Autodesk Inventor part; units mm, degrees
(part 3 of 3)
  spline S315 degree 2 poles (6.6876, 44.1549) (5.7783, 44.1549) (4.927, 45.5678) (4.927, 47.0164) knots 0 0 0 1 2 2 2
  spline S316 degree 2 poles (4.927, 47.0164) (4.927, 48.505) (5.7872, 49.8823) (6.6876, 49.8823) knots 0 0 0 1 2 2 2
  spline S317 degree 2 poles (6.6876, 49.8823) (7.5923, 49.8823) (8.4436, 48.456) (8.4436, 47.0208) knots 0 0 0 1 2 2 2
  spline S318 degree 2 poles (7.4987, 45.345) (7.6057, 45.6169) (7.6949, 46.4548) (7.6949, 47.0208) knots 0 0 0 1 2 2 2
  spline S319 degree 2 poles (7.6949, 47.0208) (7.6949, 47.5869) (7.6057, 48.4203) (7.4943, 48.7011) knots 0 0 0 1 2 2 2
  spline S320 degree 2 poles (7.4943, 48.7011) (7.3829, 48.9819) (6.9951, 49.2716) (6.6876, 49.2716) knots 0 0 0 1 2 2 2
  spline S321 degree 2 poles (6.6876, 49.2716) (6.38, 49.2716) (5.9833, 48.9819) (5.8675, 48.6922) knots 0 0 0 1 2 2 2
  spline S322 degree 2 poles (5.8675, 48.6922) (5.756, 48.4114) (5.6758, 47.5557) (5.6758, 47.0164) knots 0 0 0 1 2 2 2
  spline S323 degree 2 poles (5.6758, 47.0164) (5.6758, 46.437) (5.7471, 45.6614) (5.863, 45.3583) knots 0 0 0 1 2 2 2
  spline S324 degree 2 poles (5.863, 45.3583) (5.97, 45.0731) (6.3667, 44.7656) (6.6876, 44.7656) knots 0 0 0 1 2 2 2
  spline S325 degree 2 poles (6.6876, 44.7656) (6.9906, 44.7656) (7.3873, 45.0553) (7.4987, 45.345) knots 0 0 0 1 2 2 2
  spline S326 degree 2 poles (4.2735, 17.0475) (4.2735, 15.5677) (3.4133, 14.1816) (2.5174, 14.1816) knots 0 0 0 1 2 2 2
  spline S327 degree 2 poles (2.5174, 14.1816) (1.6082, 14.1816) (0.7569, 15.5945) (0.7569, 17.043) knots 0 0 0 1 2 2 2
  spline S328 degree 2 poles (0.7569, 17.043) (0.7569, 18.5317) (1.6171, 19.9089) (2.5174, 19.9089) knots 0 0 0 1 2 2 2
  spline S329 degree 2 poles (2.5174, 19.9089) (3.4222, 19.9089) (4.2735, 18.4826) (4.2735, 17.0475) knots 0 0 0 1 2 2 2
  spline S330 degree 2 poles (3.3286, 15.3716) (3.4356, 15.6435) (3.5247, 16.4814) (3.5247, 17.0475) knots 0 0 0 1 2 2 2
  spline S331 degree 2 poles (3.5247, 17.0475) (3.5247, 17.6135) (3.4356, 18.447) (3.3241, 18.7278) knots 0 0 0 1 2 2 2
  spline S332 degree 2 poles (3.3241, 18.7278) (3.2127, 19.0086) (2.825, 19.2983) (2.5174, 19.2983) knots 0 0 0 1 2 2 2
  spline S333 degree 2 poles (2.5174, 19.2983) (2.2099, 19.2983) (1.8132, 19.0086) (1.6973, 18.7188) knots 0 0 0 1 2 2 2
  spline S334 degree 2 poles (1.6973, 18.7188) (1.5859, 18.4381) (1.5057, 17.5823) (1.5057, 17.043) knots 0 0 0 1 2 2 2
  spline S335 degree 2 poles (1.5057, 17.043) (1.5057, 16.4636) (1.577, 15.6881) (1.6929, 15.385) knots 0 0 0 1 2 2 2
  spline S336 degree 2 poles (1.6929, 15.385) (1.7998, 15.0997) (2.1965, 14.7922) (2.5174, 14.7922) knots 0 0 0 1 2 2 2
  spline S337 degree 2 poles (2.5174, 14.7922) (2.8205, 14.7922) (3.2172, 15.0819) (3.3286, 15.3716) knots 0 0 0 1 2 2 2
  line L203 (4.3195, 33.9241) -> (0.9276, 33.9241)
  line L204 (0.9276, 33.9241) -> (0.9276, 34.7041)
  spline S338 degree 2 poles (0.9276, 34.7041) (1.2931, 35.0472) (1.9438, 35.6846) (2.2558, 36.0278) knots 0 0 0 1 2 2 2
  spline S339 degree 2 poles (2.2558, 36.0278) (2.8843, 36.7186) (3.3434, 37.5477) (3.3434, 37.9889) knots 0 0 0 1 2 2 2
  spline S340 degree 2 poles (3.3434, 37.9889) (3.3434, 38.2207) (3.2007, 38.5683) (3.0715, 38.6797) knots 0 0 0 1 2 2 2
  spline S341 degree 2 poles (3.0715, 38.6797) (2.9422, 38.7912) (2.6035, 38.9026) (2.3985, 38.9026) knots 0 0 0 1 2 2 2
  spline S342 degree 2 poles (2.3985, 38.9026) (2.2024, 38.9026) (1.8012, 38.8045) (1.6185, 38.7288) knots 0 0 0 1 2 2 2
  spline S343 degree 2 poles (1.6185, 38.7288) (1.4625, 38.6664) (1.1728, 38.4881) (1.0836, 38.4257) knots 0 0 0 1 2 2 2
  line L205 (1.0836, 38.4257) -> (1.0435, 38.4257)
  line L206 (1.0435, 38.4257) -> (1.0435, 39.2101)
  spline S344 degree 2 poles (1.0435, 39.2101) (1.2708, 39.3216) (2.0865, 39.54) (2.452, 39.54) knots 0 0 0 1 2 2 2
  spline S345 degree 2 poles (2.452, 39.54) (3.223, 39.54) (4.0921, 38.7243) (4.0921, 38.029) knots 0 0 0 1 2 2 2
  spline S346 degree 2 poles (4.0921, 38.029) (4.0921, 37.7037) (3.9406, 37.1599) (3.8069, 36.9281) knots 0 0 0 1 2 2 2
  spline S347 degree 2 poles (3.8069, 36.9281) (3.6732, 36.6874) (3.2854, 36.215) (3.0715, 35.9877) knots 0 0 0 1 2 2 2
  spline S348 degree 2 poles (3.0715, 35.9877) (2.7238, 35.6088) (1.8725, 34.7977) (1.6185, 34.5614) knots 0 0 0 1 2 2 2
  line L207 (1.6185, 34.5614) -> (4.3195, 34.5614)
  line L208 (4.3195, 34.5614) -> (4.3195, 33.9241)
  spline S349 degree 2 poles (8.4779, 36.6741) (8.4779, 35.1943) (7.6177, 33.8082) (6.7218, 33.8082) knots 0 0 0 1 2 2 2
  spline S350 degree 2 poles (6.7218, 33.8082) (5.8126, 33.8082) (4.9613, 35.2211) (4.9613, 36.6696) knots 0 0 0 1 2 2 2
  spline S351 degree 2 poles (4.9613, 36.6696) (4.9613, 38.1583) (5.8215, 39.5355) (6.7218, 39.5355) knots 0 0 0 1 2 2 2
  spline S352 degree 2 poles (6.7218, 39.5355) (7.6266, 39.5355) (8.4779, 38.1092) (8.4779, 36.6741) knots 0 0 0 1 2 2 2
  spline S353 degree 2 poles (7.533, 34.9982) (7.64, 35.2701) (7.7291, 36.108) (7.7291, 36.6741) knots 0 0 0 1 2 2 2
  spline S354 degree 2 poles (7.7291, 36.6741) (7.7291, 37.2401) (7.64, 38.0736) (7.5285, 38.3544) knots 0 0 0 1 2 2 2
  spline S355 degree 2 poles (7.5285, 38.3544) (7.4171, 38.6352) (7.0293, 38.9249) (6.7218, 38.9249) knots 0 0 0 1 2 2 2
  spline S356 degree 2 poles (6.7218, 38.9249) (6.4143, 38.9249) (6.0176, 38.6352) (5.9017, 38.3455) knots 0 0 0 1 2 2 2
  spline S357 degree 2 poles (5.9017, 38.3455) (5.7903, 38.0647) (5.7101, 37.2089) (5.7101, 36.6696) knots 0 0 0 1 2 2 2
  spline S358 degree 2 poles (5.7101, 36.6696) (5.7101, 36.0902) (5.7814, 35.3147) (5.8973, 35.0116) knots 0 0 0 1 2 2 2
  spline S359 degree 2 poles (5.8973, 35.0116) (6.0042, 34.7263) (6.4009, 34.4188) (6.7218, 34.4188) knots 0 0 0 1 2 2 2
  spline S360 degree 2 poles (6.7218, 34.4188) (7.0249, 34.4188) (7.4216, 34.7085) (7.533, 34.9982) knots 0 0 0 1 2 2 2
  point P0 (190.5653, 91.5)
  point P1 (8.4853, 17.25)
  dimension "d94" = 1
  constraints: 14 end point, 3 midpoint, 2 parallel, 2 perpendicular, 2 point on line, 1 horizontal, 30 other
  measures "d94" distance of L61.end L62.end
extrude "Extrusion14" add sketch "Skizze14" along normal blind 1 contours L61 L62 L63 L67 | L68 L69 L70 L71 L72 L73 S0 L74 L75 L76 L77 | S1 S2 S3 S4 S5 S6 S7 L78 L79 S8 S9 S10 S11 S12 | S20 S21 S22 S23 | L80 L81 L82 L83 L84 L85 S32 L86 L87 L88 L89 | S33 S34 S35 L90 L91 S36 S37 S38 S39 S40 S41 S42 L92 L93 L94 L95 L96 S43 S44 S45 | S46 S47 S48 S49 | L97 L98 L99 L100 L101 L102 S58 L103 L104 L105 L106 | S59 S60 L107 L108 S61 S62 S63 S64 L109 S65 S66 S67 S68 S69 L110 L111 S70 S71 S72 S73 S74 L112 L113 L114 S75 S76 S77 | S78 S79 S80 S81 | L115 L116 L117 L118 L119 L120 S90 L121 L122 L123 L124 | L125 L126 S91 S92 S93 S94 S95 S96 L127 L128 S97 S98 S99 S100 S101 L129 L130 | S102 S103 S104 S105 | L131 L132 L133 L134 L135 L136 S114 L137 L138 L139 L140 | L141 L142 L143 L144 L145 L146 S115 L147 L148 L149 L150 | S116 S117 S118 S119 | L151 L152 L153 L154 L155 L156 S128 L157 L158 L159 L160 | S129 S130 S131 S132 | S141 S142 S143 S144 | S153 S154 S155 S156 S157 S158 S159 L161 L162 S160 S161 S162 S163 S164 | S172 S173 S174 S175 | S184 S185 S186 L163 S187 S188 S189 S190 L164 S191 S192 | S203 S204 S205 S206 | L165 L166 L167 L168 L169 L170 L171 | S215 S216 S217 S218 | S227 S228 S229 S230 S231 S232 S233 L172 L173 S234 S235 S236 S237 S238 | S246 S247 S248 S249 | S258 S259 S260 L174 L175 S261 S262 S263 S264 S265 S266 S267 L176 L177 L178 L179 L180 S268 S269 S270 | S271 S272 S273 S274 | L181 L182 L183 L184 L185 L186 L187 L188 L189 L190 L191 | S283 S284 S285 S286 | S295 S296 L195 L196 S297 S298 S299 S300 L197 S301 S302 S303 S304 S305 L198 L199 S306 S307 S308 S309 S310 L200 L201 L202 S311 S312 S313 | S314 S315 S316 S317 | S326 S327 S328 S329 | L203 L204 S338 S339 S340 S341 S342 S343 L205 L206 S344 S345 S346 S347 S348 L207 L208 | S349 S350 S351 S352
sketch "Skizze17" plane through (-65, -62, 24) normal (0, -1, 0) x (1, 0, 0)
  line L0 (-5, 0) -> (-5, 156.5)
  line L1 (-5, 156.5) -> (-6, 157.5) projected
  line L2 (-5, 156.5) -> (-6, 157.5)
  line L3 (-13.5, 165) -> (-22, 156.5) projected
  line L4 (-6, 157.5) -> (-13.5, 165)
  line L5 (-13.5, 165) -> (-22, 156.5)
  line L6 (-5, 0) -> (-22, 0) projected
  line L7 (-22, 156.5) -> (-22, 0)
  line L8 (-22, 0) -> (-5, 0)
  line L9 (135, 0) -> (135, 156.5)
  line L10 (136, 157.4) -> (135, 156.5) projected
  line L11 (135, 156.5) -> (136, 157.4)
  line L12 (143.9474, 164.5526) -> (136, 157.4) projected
  line L13 (136, 157.4) -> (143.9474, 164.5526)
  line L14 (152, 0) -> (152, 156.5) projected
  line L15 (143.9474, 164.5526) -> (152, 156.5)
  line L16 (136, 0) -> (152, 0) projected
  line L17 (152, 156.5) -> (152, 0)
  line L18 (152, 0) -> (135, 0)
  point P0 (65, -24)
  constraints: 25 end point, 4 collinear, 4 perpendicular, 1 vertical
extrude "Extrusion15" add sketch "Skizze17" against normal blind 3
sketch "Skizze18" plane through (-71, -86.5, 181.5) normal (1, 0, 0) x (0, 0, -1)
  line L0 (-5, 24.5) -> (1, 24.5) projected
  line L1 (0, 24.5) -> (0, 0) projected
  line L2 (0, 24.5) -> (0, 0)
  line L3 (157.5, 0) -> (160.5, 0) projected
  line L4 (0, 0) -> (157.5, 0)
  line L5 (157.5, 24.5) -> (160.5, 24.5) projected
  line L6 (157.5, 0) -> (157.5, 24.5)
  line L7 (-5, 24.5) -> (0, 24.5) projected
  line L8 (157.5, 24.5) -> (0, 24.5)
  point P0 (181.5, 86.5)
  point P1 (1, 24.5)
  constraints: 8 end point, 3 collinear, 1 perpendicular, 1 point on line
extrude "Extrusion16" add sketch "Skizze18" against normal blind 3
sketch "Skizze20" plane through (71, -86.5, 181.4) normal (-1, 0, 0) x (0, 0, 1)
  line L0 (5.1, 24.5) -> (0, 24.5) projected
  line L1 (0, 0) -> (0, 24.5) projected
  line L2 (0, 24.5) -> (0, 0)
  line L3 (-157.4, 0) -> (-157.4, 24.5) projected
  line L4 (0, 0) -> (-157.4, 0)
  line L5 (-157.4, 0) -> (-157.4, 24.5)
  line L6 (-157.4, 24.5) -> (0, 24.5)
  point P0 (-181.4, 86.5)
  constraints: 8 end point, 3 perpendicular, 1 collinear
extrude "Extrusion17" add sketch "Skizze20" against normal blind 3
sketch "Skizze30" plane through (89, -91.5, 0) normal (1, 0, 0) x (0, 0, -1)
  line L0 (0, 0) -> (0, 183) projected
  line L1 (-24, 181) -> (-24, 32.5) projected
  line L2 (0, 183) -> (-24, 183)
  line L3 (-24, 183) -> (-24, 159)
  line L4 (-24, 159) -> (0, 159)
  line L5 (0, 159) -> (0, 183)
  line L6 (-180.5, 183) -> (-180.5, 169.25) projected
  line L7 (-180.5, 183) -> (-156.5, 183)
  line L8 (-156.5, 183) -> (-156.5, 159)
  line L9 (-156.5, 159) -> (-180.5, 159)
  line L10 (-180.5, 159) -> (-180.5, 183)
  line L11 (-24, 0) -> (-180.5, 0) projected
  line L12 (-180.5, 0) -> (-156.5, 0)
  line L13 (-156.5, 0) -> (-156.5, 24)
  line L14 (-156.5, 24) -> (-180.5, 24)
  line L15 (-180.5, 24) -> (-180.5, 0)
  line L16 (0, 0) -> (-24, 0)
  line L17 (-24, 0) -> (-24, 24)
  line L18 (-24, 24) -> (0, 24)
  line L19 (0, 24) -> (0, 0)
  point P0 (0, 91.5)
  point P1 (0, 24)
  dimension "d140" = 24
  dimension "d141" = 24
  dimension "d142" = 24
  dimension "d143" = 24
  dimension "d144" = 24
  dimension "d145" = 24
  dimension "d146" = 24
  constraints: 32 end point, 8 parallel, 4 horizontal, 4 perpendicular, 1 point on line
  measures "d140" distance of L0.end L2.end
  measures "d141" distance of L3.end L2.end
  measures "d142" distance of L6.start L7.end
  measures "d143" distance of L13.end L14.end
  measures "d144" distance of L12.end L13.end
  measures "d145" distance of L17.end L18.end
  measures "d146" distance of L16.end L17.end
extrude "Extrusion20" add sketch "Skizze30" against normal blind 5
sketch "Skizze33" plane through (89, -91.5, 0) normal (1, 0, 0) x (0, 0, -1)
  line L0 (-180.5, 0) -> (-180.5, 183) projected
  line L1 (0, 0) -> (-180.5, 0) projected
  line L2 (0, 183) -> (-180.5, 183) projected
  line L3 (0, 183) -> (-180.5, 183) projected
  line L4 (0, 0) -> (0, 183) projected
  line L5 (-5, 5) -> (-19, 5)
  line L6 (-19, 5) -> (-19, 19)
  line L7 (-19, 19) -> (-5, 19)
  line L8 (-5, 19) -> (-5, 5)
  line L9 (-5, 178) -> (-19, 178)
  line L10 (-19, 178) -> (-19, 164)
  line L11 (-19, 164) -> (-5, 164)
  line L12 (-5, 164) -> (-5, 178)
  line L13 (-175.5, 178) -> (-161.5, 178)
  line L14 (-161.5, 178) -> (-161.5, 164)
  line L15 (-161.5, 164) -> (-175.5, 164)
  line L16 (-175.5, 164) -> (-175.5, 178)
  line L17 (-175.5, 5) -> (-161.5, 5)
  line L18 (-161.5, 5) -> (-161.5, 19)
  line L19 (-161.5, 19) -> (-175.5, 19)
  line L20 (-175.5, 19) -> (-175.5, 5)
  point P0 (0, 91.5)
  point P1 (-32, 183)
  point P2 (-31, 183)
  dimension "d161" = 5
  dimension "d162" = 5
  dimension "d163" = 5
  dimension "d164" = 5
  dimension "d165" = 5
  dimension "d166" = 5
  dimension "d167" = 5
  dimension "d168" = 5
  dimension "d169" = 14
  dimension "d170" = 14
  dimension "d171" = 14
  dimension "d172" = 14
  dimension "d173" = 14
  dimension "d174" = 14
  dimension "d175" = 14
  dimension "d176" = 14
  constraints: 32 end point, 8 parallel, 4 horizontal, 4 perpendicular, 2 point on line
  measures "d161" distance from line of L17.start L0
  measures "d162" distance from line of L1 L17.start
  measures "d163" distance from line of L2 L13.start
  measures "d164" distance from line of L13.start L0
  measures "d165" distance from line of L3 L9.start
  measures "d166" distance from line of L9.start L4
  measures "d167" distance from line of L5.start L1
  measures "d168" distance from line of L5.start L4
  measures "d169" distance of L19.end L17.start
  measures "d170" distance of L18.end L19.end
  measures "d171" distance of L14.end L15.end
  measures "d172" distance of L15.end L13.start
  measures "d173" distance of L9.end L10.end
  measures "d174" distance of L9.start L9.end
  measures "d175" distance of L6.end L7.end
  measures "d176" distance of L5.end L6.end
extrude "Extrusion21" cut sketch "Skizze33" against normal blind 3 contours L5 L6 L7 L8 | L12 L11 L10 L9 | L13 L14 L15 L16 | L20 L19 L18 L17
sketch "Skizze35" plane through (-89, 91.5, 0) normal (0, 1, 0) x (1, 0, 0)
  line L0 (154, -24) -> (24, -24) projected
  line L1 (79, 24) -> (99, 24)
  line L2 (99, 24) -> (99, -24)
  line L3 (99, -24) -> (79, -24)
  line L4 (79, -24) -> (79, 24)
  line L5 (79, 24) -> (99, -24) construction
  line L6 (99, 24) -> (79, -24) construction
  line L7 (78, -24) -> (80, -24)
  line L8 (80, -24) -> (80, 24)
  line L9 (80, 24) -> (78, 24)
  line L10 (78, 24) -> (78, -24)
  line L11 (78, -24) -> (80, 24) construction
  line L12 (80, -24) -> (78, 24) construction
  line L13 (100, -24) -> (98, -24)
  line L14 (98, -24) -> (98, 24)
  line L15 (98, 24) -> (100, 24)
  line L16 (100, 24) -> (100, -24)
  line L17 (13.65, 0) -> (164.35, 0) projected
  line L18 (100, -24) -> (98, 24) construction
  line L19 (98, -24) -> (100, 24) construction
  point P0 (89, 0)
  point P1 (79, 0)
  point P2 (99, 0)
  point P3 (78, 0)
  point P4 (100, 0)
  dimension "d179" = 20
  dimension "d180" = 2
  dimension "d181" = 2
  constraints: 36 end point, 8 midpoint, 6 parallel, 4 point on line, 3 horizontal, 3 perpendicular
  measures "d179" distance of L1.start L1.end
  measures "d180" distance of L14.end L15.end
  measures "d181" distance of L9.end L8.end
extrude "Extrusion22" cut sketch "Skizze35" against normal blind 1 contours L0 L2 L17 L16 | L0 L10 L17 L4
sketch "Skizze36" plane through (-89, 90.5, 0) normal (0, 1, 0) x (1, 0, 0)
  line L0 (78, -24) -> (78, 0) projected
  line L1 (78, 0) -> (79, 0)
  line L2 (79, 0) -> (79, -1)
  line L3 (79, -1) -> (78, -1)
  line L4 (78, -1) -> (78, 0)
  line L5 (13.65, 0) -> (164.35, 0) projected
  line L6 (99, 0) -> (100, 0)
  line L7 (100, 0) -> (100, -1)
  line L8 (100, -1) -> (99, -1)
  line L9 (99, -1) -> (99, 0)
  point P0 (89, 0)
  constraints: 16 end point, 4 parallel, 2 horizontal, 2 perpendicular, 1 point on line
extrude "Extrusion23" cut sketch "Skizze36" against normal blind 20
sketch "Skizze38" plane through (-89, 91.5, 180.5) normal (0, 1, 0) x (1, 0, 0)
  line L0 (24, 156.5) -> (24, 92) projected
  line L1 (154, 156.5) -> (154, 92) projected
  point P0 (89, 180.5)
  dimension "d186" = 130
  measures "d186" distance between parallel lines of L0 L1
sketch "Skizze39" plane through (0, 0, 24) normal (0, 0, 1) x (1, 0, 0)
  circle A0 centre (-60.35, 54) radius 1.7 projected
  circle A1 centre (-60.35, 54) radius 3
  circle A2 centre (0, 54) radius 1.7 projected
  circle A3 centre (0, 54) radius 3
  circle A4 centre (60.35, 54) radius 1.7 projected
  circle A5 centre (60.35, 54) radius 3
  circle A6 centre (60.35, 2.5) radius 1.7 projected
  circle A7 centre (60.35, 2.5) radius 3
  circle A8 centre (-60.35, 2.5) radius 1.7 projected
  circle A9 centre (-60.35, 2.5) radius 3
  circle A10 centre (-60.35, -49) radius 1.7 projected
  circle A11 centre (-60.35, -49) radius 3
  circle A12 centre (0, -49) radius 1.7 projected
  circle A13 centre (0, -49) radius 3
  circle A14 centre (60.35, -49) radius 1.7 projected
  circle A15 centre (60.35, -49) radius 3
  point P0 (0, 0)
  dimension "d188" = 6
  dimension "d189" = 6
  dimension "d190" = 6
  dimension "d191" = 6
  dimension "d192" = 6
  dimension "d193" = 6
  dimension "d194" = 6
  dimension "d195" = 6
  constraints: 8 centre point, 8 coincident
  measures "d188" diameter of A15
  measures "d189" diameter of A13
  measures "d190" diameter of A11
  measures "d191" diameter of A9
  measures "d192" diameter of A1
  measures "d193" diameter of A3
  measures "d194" diameter of A5
  measures "d195" diameter of A7
extrude "Extrusion24" cut sketch "Skizze39" against normal blind 20 contours A0 | A1 | A3 | A4 | A5 | A6 | A7 | A8 | A9 | A11 | A12 | A13 | A14 | A15
sketch "Skizze40" plane through (0, 0, 0) normal (0, 0, -1) x (-1, 0, 0)
  line L0 (-89, -91.5) -> (-89, 91.5) projected
  line L1 (89, 91.5) -> (89, -91.5) projected
  line L2 (-89, 91.5) -> (89, 91.5)
  line L3 (89, 91.5) -> (89, -91.5)
  line L4 (89, -91.5) -> (-89, -91.5)
  line L5 (-89, -91.5) -> (-89, 91.5)
  point P0 (0, 0)
  constraints: 8 end point, 2 parallel, 1 horizontal, 1 perpendicular
extrude "Extrusion25" cut sketch "Skizze40" against normal blind 24
sketch "Skizze41" plane through (77, 91.5, 192.5) normal (0, 0, -1) x (0, -1, 0)
  line L0 (0, 166) -> (0, 154) projected
  line L1 (183, 12) -> (183, -12) projected
  line L2 (0, 166) -> (183, 166)
  line L3 (183, 166) -> (183, -12)
  line L4 (183, -12) -> (0, -12)
  line L5 (0, -12) -> (0, 166)
  point P0 (91.5, 77)
  constraints: 8 end point, 2 parallel, 1 horizontal, 1 perpendicular
extrude "Extrusion26" cut sketch "Skizze41" against normal mid plane 24
sketch "Skizze42" plane through (0, 0, 24) normal (0, 0, -1) x (-1, 0, 0)
  line L0 (-87, 89.5) -> (-70, 89.5) projected
  line L1 (-70, -59) -> (-87, -59) projected
  line L2 (-87, 89.5) -> (-70, 89.5)
  line L3 (-70, 89.5) -> (-70, -59)
  line L4 (-70, -59) -> (-87, -59)
  line L5 (-87, -59) -> (-87, 89.5)
  line L6 (-87, -62) -> (-87, -67.5) projected
  line L7 (-74, -62) -> (-74, -86.5) projected
  line L8 (-87, -62) -> (-74, -62)
  line L9 (-74, -62) -> (-74, -86.5)
  line L10 (-74, -86.5) -> (-87, -86.5)
  line L11 (-87, -86.5) -> (-87, -62)
  line L12 (74, -86.5) -> (74, -62) projected
  line L13 (87, -86.5) -> (87, -62) projected
  line L14 (74, -62) -> (87, -62)
  line L15 (87, -62) -> (87, -86.5)
  line L16 (87, -86.5) -> (74, -86.5)
  line L17 (74, -86.5) -> (74, -62)
  line L18 (70, 89.5) -> (70, -59) projected
  line L19 (87, -59) -> (70, -59) projected
  line L20 (70, 89.5) -> (87, 89.5)
  line L21 (87, 89.5) -> (87, -59)
  line L22 (87, -59) -> (70, -59)
  line L23 (70, -59) -> (70, 89.5)
  point P0 (0, 0)
  constraints: 32 end point, 8 parallel, 4 horizontal, 4 perpendicular
extrude "Extrusion27" add sketch "Skizze42" against normal up to surface (156.5 mm away)
sketch "Skizze43" plane through (89, -91.5, 180.5) normal (1, 0, 0) x (0, 0, -1)
  line L0 (5, 178) -> (19, 178) projected
  line L1 (5, 178) -> (19, 178)
  line L2 (19, 178) -> (19, 164)
  line L3 (19, 164) -> (5, 164)
  line L4 (5, 164) -> (5, 178)
  line L5 (5, 5) -> (5, 19) projected
  line L6 (2, 5) -> (26.5, 5) projected
  line L7 (5, 19) -> (19, 19)
  line L8 (19, 19) -> (19, 5)
  line L9 (19, 5) -> (5, 5)
  line L10 (5, 5) -> (5, 19)
  point P0 (180.5, 91.5)
  constraints: 16 end point, 4 parallel, 2 horizontal, 2 perpendicular, 2 point on line
extrude "Extrusion28" cut sketch "Skizze43" against normal blind 3
ref_plane "Arbeitsebene2" through (0, 0, 29) normal (0, 0, -1) x (-1, 0, 0)
sketch "Skizze44" plane through (0, 0, 29) normal (0, 0, -1) x (-1, 0, 0)
  line L0 (-84.85, 73.1454) -> (-82, 74.7909)
  line L1 (-84.85, 69.8546) -> (-84.85, 73.1454)
  line L2 (-82, 74.7909) -> (-79.15, 73.1454)
  line L3 (-82, 68.2091) -> (-84.85, 69.8546)
  line L4 (-79.15, 73.1454) -> (-79.15, 69.8546)
  line L5 (-79.15, 69.8546) -> (-82, 68.2091)
  line L6 (-82, 74.7909) -> (-96.75, 74.7909)
  line L7 (-82, 68.2091) -> (-96.75, 68.2091)
  line L8 (-96.75, 74.7909) -> (-96.75, 68.2091)
  line L9 (-89, 91.5) -> (-65, 91.5) construction
  line L10 (-82, 91.5) -> (-82, -91.5) construction
  line L11 (-65, -91.5) -> (-89, -91.5) construction
  line L12 (-89, -91.5) -> (-89, 91.5) construction
  line L13 (-65, -62) -> (-65, 91.5) construction
  line L14 (-79.15, 33.1454) -> (-79.15, 29.8546)
  line L15 (-82, 34.7909) -> (-79.15, 33.1454)
  line L16 (-79.15, 29.8546) -> (-82, 28.2091)
  line L17 (-82, 28.2091) -> (-84.85, 29.8546)
  line L18 (-84.85, 29.8546) -> (-84.85, 33.1454)
  line L19 (-84.85, 33.1454) -> (-82, 34.7909)
  line L20 (-82, 34.7909) -> (-96.75, 34.7909)
  line L21 (-82, 28.2091) -> (-96.75, 28.2091)
  line L22 (-96.75, 34.7909) -> (-96.75, 28.2091)
  line L23 (-82, -8.2091) -> (-79.15, -9.8546)
  line L24 (-79.15, -9.8546) -> (-79.15, -13.1454)
  line L25 (-79.15, -13.1454) -> (-82, -14.7909)
  line L26 (-82, -14.7909) -> (-84.85, -13.1454)
  line L27 (-84.85, -9.8546) -> (-82, -8.2091)
  line L28 (-84.85, -13.1454) -> (-84.85, -9.8546)
  line L29 (-82, -14.7909) -> (-96.75, -14.7909)
  line L30 (-82, -8.2091) -> (-96.75, -8.2091)
  line L31 (-96.75, -8.2091) -> (-96.75, -14.7909)
  line L32 (-82, -48.2091) -> (-79.15, -49.8546)
  line L33 (-79.15, -49.8546) -> (-79.15, -53.1454)
  line L34 (-79.15, -53.1454) -> (-82, -54.7909)
  line L35 (-82, -54.7909) -> (-84.85, -53.1454)
  line L36 (-84.85, -49.8546) -> (-82, -48.2091)
  line L37 (-84.85, -53.1454) -> (-84.85, -49.8546)
  line L38 (-82, -54.7909) -> (-96.75, -54.7909)
  line L39 (-82, -48.2091) -> (-96.75, -48.2091)
  line L40 (-96.75, -48.2091) -> (-96.75, -54.7909)
  line L41 (0, 91.5) -> (0, -95.2854)
  line L42 (79.15, 73.1454) -> (79.15, 69.8546)
  line L43 (82, 74.7909) -> (79.15, 73.1454)
  line L44 (79.15, 69.8546) -> (82, 68.2091)
  line L45 (82, 68.2091) -> (84.85, 69.8546)
  line L46 (84.85, 69.8546) -> (84.85, 73.1454)
  line L47 (84.85, 73.1454) -> (82, 74.7909)
  line L48 (82, 74.7909) -> (96.75, 74.7909)
  line L49 (82, 68.2091) -> (96.75, 68.2091)
  line L50 (96.75, 74.7909) -> (96.75, 68.2091)
  line L51 (94, 91.5) -> (70, 91.5) construction
  line L52 (82, 91.5) -> (82, -91.5) construction
  line L53 (70, -91.5) -> (94, -91.5) construction
  line L54 (94, -91.5) -> (94, 91.5) construction
  line L55 (70, -62) -> (70, 91.5) construction
  line L56 (82, 34.7909) -> (79.15, 33.1454)
  line L57 (79.15, 33.1454) -> (79.15, 29.8546)
  line L58 (79.15, 29.8546) -> (82, 28.2091)
  line L59 (82, 28.2091) -> (84.85, 29.8546)
  line L60 (84.85, 33.1454) -> (82, 34.7909)
  line L61 (84.85, 29.8546) -> (84.85, 33.1454)
  line L62 (82, 28.2091) -> (96.75, 28.2091)
  line L63 (82, 34.7909) -> (96.75, 34.7909)
  line L64 (96.75, 34.7909) -> (96.75, 28.2091)
  line L65 (82, -14.7909) -> (84.85, -13.1454)
  line L66 (82, -8.2091) -> (96.75, -8.2091)
  line L67 (82, -8.2091) -> (79.15, -9.8546)
  line L68 (84.85, -9.8546) -> (82, -8.2091)
  line L69 (96.75, -8.2091) -> (96.75, -14.7909)
  line L70 (82, -14.7909) -> (96.75, -14.7909)
  line L71 (84.85, -13.1454) -> (84.85, -9.8546)
  line L72 (79.15, -9.8546) -> (79.15, -13.1454)
  line L73 (79.15, -13.1454) -> (82, -14.7909)
  line L74 (82, -54.7909) -> (84.85, -53.1454)
  line L75 (82, -48.2091) -> (96.75, -48.2091)
  line L76 (82, -48.2091) -> (79.15, -49.8546)
  line L77 (84.85, -49.8546) -> (82, -48.2091)
  line L78 (96.75, -48.2091) -> (96.75, -54.7909)
  line L79 (82, -54.7909) -> (96.75, -54.7909)
  line L80 (84.85, -53.1454) -> (84.85, -49.8546)
  line L81 (79.15, -49.8546) -> (79.15, -53.1454)
  line L82 (79.15, -53.1454) -> (82, -54.7909)
  circle A0 centre (82, 71.5) radius 1.7
  circle A1 centre (82, 31.5) radius 1.7
  circle A2 centre (82, -11.5) radius 1.7
  circle A3 centre (82, -51.5) radius 1.7
  circle A4 centre (-82, -51.5) radius 1.7
  circle A5 centre (-82, -11.5) radius 1.7
  circle A6 centre (-82, 31.5) radius 1.7
  circle A7 centre (-82, 71.5) radius 1.7
  point P0 (0, 0)
  point P1 (-82, 71.5)
  point P2 (-82, 71.5)
  point P3 (-82, -51.5)
  point P4 (-82, -11.5)
  point P5 (-82, 31.5)
  point P6 (-82, -11.5)
  point P7 (-82, -11.5)
  point P8 (-82, -11.5)
  point P9 (-82, -51.5)
  point P10 (82, 71.5)
  point P11 (82, -51.5)
  point P12 (82, -11.5)
  point P13 (82, 31.5)
  point P14 (82, -11.5)
  point P15 (82, -11.5)
  point P16 (82, -11.5)
  point P17 (82, -51.5)
  point P18 (82, -51.5)
  point P19 (82, -51.5)
  point P20 (82, 31.5)
  point P21 (82, -11.5)
  point P22 (82, -51.5)
  point P23 (-82, -51.5)
  point P24 (-82, -11.5)
  point P25 (-82, 31.5)
  point P26 (-82, 71.5)
  point P27 (-82, 71.5)
  dimension "d207" = 5.7
  dimension "d208" = 7
  dimension "d209" = 17
  dimension "d210" = 20
  dimension "d211" = 40
  dimension "d212" = 40
  dimension "d213" = 40
  dimension "d214" = 5.7
  dimension "d215" = 5.7
  dimension "d216" = 5.7
  dimension "d225" = 3.4
  dimension "d226" = 3.4
  dimension "d227" = 3.4
  dimension "d228" = 3.4
  dimension "d229" = 3.4
  dimension "d230" = 3.4
  dimension "d231" = 3.4
  dimension "d232" = 3.4
  dimension "d253" = 0
  dimension "d254" = 0
  constraints: 158 end point, 8 centre point, 8 point on line, 1 coincident, 1 midpoint, 1 parallel, 1 vertical, 52 other
  measures "d207" distance between parallel lines of L4 L1
  measures "d208" distance between parallel lines of L12 L10
  measures "d209" distance between parallel lines of L10 L13
  measures "d210" distance from line of L9 point (-82, 71.5)
  measures "d211" distance of L10.end point (-82, -51.5)
  measures "d212" distance of point (-82, 31.5) point (-82, 71.5)
  measures "d213" distance of point (-82, -51.5) point (-82, -11.5)
  measures "d214" distance between parallel lines of L14 L18
  measures "d215" distance between parallel lines of L24 L28
  measures "d216" distance between parallel lines of L33 L37
  measures "d225" diameter of A0
  measures "d226" diameter of A1
  measures "d227" diameter of A2
  measures "d228" diameter of A3
  measures "d229" diameter of A4
  measures "d230" diameter of A5
  measures "d231" diameter of A6
  measures "d232" diameter of A7
  measures "d253" distance of point (-82, 71.5) point (-82, 71.5)
  measures "d254" distance of point (82, 71.5) point (82, 71.5)
extrude "Extrusion29" cut sketch "Skizze44" against normal blind 2.6 contours L1 L3 L7 L8 L6 L0 | L0 L2 L4 L5 L3 L1 | L14 L16 L17 L18 L19 L15 | L19 L18 L17 L21 L22 L20 | L23 L24 L25 L26 L28 L27 | L27 L28 L26 L29 L31 L30 | L32 L33 L34 L35 L37 L36 | L36 L37 L35 L38 L40 L39 | L43 L47 L46 L45 L44 L42 | L48 L50 L49 L45 L46 L47 | L60 L61 L59 L58 L57 L56 | L63 L64 L62 L59 L61 L60 | L73 L72 L67 L68 L71 L65 | L65 L71 L68 L66 L69 L70 | L82 L81 L76 L77 L80 L74 | L74 L80 L77 L75 L78 L79 | A0 | A1 | A2 | A3 | A4 | A5 | A6 | A7
sketch "Skizze45" plane through (89, -91.5, 180.5) normal (1, 0, 0) x (0, 0, -1)
  line L0 (148.9, 166.2909) -> (151.5, 166.2909) construction
  line L1 (151.5, 159.7091) -> (148.9, 159.7091) construction
  line L2 (148.9, 166.2909) -> (151.5, 159.7091) construction
  line L3 (151.5, 159.7091) -> (151.5, 166.2909) construction
  line L4 (151.5, 166.2909) -> (148.9, 159.7091) construction
  line L5 (148.9, 126.2909) -> (148.9, 124.6454) construction
  line L6 (151.5, 119.7091) -> (148.9, 119.7091) construction
  line L7 (148.9, 126.2909) -> (151.5, 119.7091) construction
  line L8 (148.9, 126.2909) -> (151.5, 126.2909) construction
  line L9 (151.5, 126.2909) -> (148.9, 119.7091) construction
  line L10 (148.9, 83.2909) -> (151.5, 83.2909) construction
  line L11 (151.5, 76.7091) -> (151.5, 78.3546) construction
  line L12 (148.9, 83.2909) -> (151.5, 76.7091) construction
  line L13 (151.5, 81.6454) -> (151.5, 83.2909) construction
  line L14 (151.5, 76.7091) -> (148.9, 76.7091) construction
  line L15 (151.5, 83.2909) -> (148.9, 76.7091) construction
  line L16 (148.9, 43.2909) -> (148.9, 41.6454) construction
  line L17 (151.5, 36.7091) -> (148.9, 36.7091) construction
  line L18 (148.9, 43.2909) -> (151.5, 36.7091) construction
  line L19 (151.5, 43.2909) -> (148.9, 43.2909) construction
  line L20 (151.5, 43.2909) -> (148.9, 36.7091) construction
  circle A0 centre (150.2, 40) radius 0.8
  circle A1 centre (150.2, 80) radius 0.8
  circle A2 centre (150.2, 123) radius 0.8
  circle A3 centre (150.2, 163) radius 0.8
  point P0 (180.5, 91.5)
  dimension "d219" = 1.6
  dimension "d220" = 1.6
  dimension "d221" = 1.6
  dimension "d222" = 1.6
  constraints: 18 end point, 4 centre point, 4 midpoint, 1 vertical
  measures "d219" diameter of A3
  measures "d220" diameter of A2
  measures "d221" diameter of A1
  measures "d222" diameter of A0
extrude "Extrusion30" cut sketch "Skizze45" against normal through all
sketch "Skizze46" plane through (0, 0, 24) normal (0, 0, -1) x (-1, 0, 0)
  line L0 (-79.15, 73.1454) -> (-79.15, 69.8546)
  line L1 (-82, 74.7909) -> (-79.15, 73.1454)
  line L2 (-79.15, 69.8546) -> (-82, 68.2091)
  line L3 (-82, 68.2091) -> (-84.85, 69.8546)
  line L4 (-84.85, 69.8546) -> (-84.85, 73.1454)
  line L5 (-84.85, 73.1454) -> (-82, 74.7909)
  line L6 (-82, 74.7909) -> (-96.75, 74.7909)
  line L7 (-82, 68.2091) -> (-96.75, 68.2091)
  line L8 (-96.75, 74.7909) -> (-96.75, 68.2091)
  line L9 (-94, 91.5) -> (-70, 91.5) construction
  line L10 (-82, 91.5) -> (-82, -91.5) construction
  line L11 (-70, -91.5) -> (-94, -91.5) construction
  line L12 (-94, -91.5) -> (-94, 91.5) construction
  line L13 (-70, -62) -> (-70, 91.5) construction
  line L14 (-82, 34.7909) -> (-79.15, 33.1454)
  line L15 (-79.15, 33.1454) -> (-79.15, 29.8546)
  line L16 (-79.15, 29.8546) -> (-82, 28.2091)
  line L17 (-82, 28.2091) -> (-84.85, 29.8546)
  line L18 (-84.85, 33.1454) -> (-82, 34.7909)
  line L19 (-84.85, 29.8546) -> (-84.85, 33.1454)
  line L20 (-82, 28.2091) -> (-96.75, 28.2091)
  line L21 (-82, 34.7909) -> (-96.75, 34.7909)
  line L22 (-96.75, 34.7909) -> (-96.75, 28.2091)
  line L23 (-82, -14.7909) -> (-84.85, -13.1454)
  line L24 (-82, -8.2091) -> (-96.75, -8.2091)
  line L25 (-82, -8.2091) -> (-79.15, -9.8546)
  line L26 (-84.85, -9.8546) -> (-82, -8.2091)
  line L27 (-96.75, -8.2091) -> (-96.75, -14.7909)
  line L28 (-82, -14.7909) -> (-96.75, -14.7909)
  line L29 (-84.85, -13.1454) -> (-84.85, -9.8546)
  line L30 (-79.15, -9.8546) -> (-79.15, -13.1454)
  line L31 (-79.15, -13.1454) -> (-82, -14.7909)
  line L32 (-82, -54.7909) -> (-84.85, -53.1454)
  line L33 (-82, -48.2091) -> (-96.75, -48.2091)
  line L34 (-82, -48.2091) -> (-79.15, -49.8546)
  line L35 (-84.85, -49.8546) -> (-82, -48.2091)
  line L36 (-96.75, -48.2091) -> (-96.75, -54.7909)
  line L37 (-82, -54.7909) -> (-96.75, -54.7909)
  line L38 (-84.85, -53.1454) -> (-84.85, -49.8546)
  line L39 (-79.15, -49.8546) -> (-79.15, -53.1454)
  line L40 (-79.15, -53.1454) -> (-82, -54.7909)
  line L41 (0, 91.5) -> (0, -95.2854)
  line L42 (79.15, 73.1454) -> (79.15, 69.8546)
  line L43 (82, 74.7909) -> (79.15, 73.1454)
  line L44 (79.15, 69.8546) -> (82, 68.2091)
  line L45 (82, 68.2091) -> (84.85, 69.8546)
  line L46 (84.85, 69.8546) -> (84.85, 73.1454)
  line L47 (84.85, 73.1454) -> (82, 74.7909)
  line L48 (82, 74.7909) -> (96.75, 74.7909)
  line L49 (96.75, 74.7909) -> (96.75, 68.2091)
  line L50 (94, 91.5) -> (70, 91.5) construction
  line L51 (82, 68.2091) -> (96.75, 68.2091)
  line L52 (82, 34.7909) -> (96.75, 34.7909)
  line L53 (82, 34.7909) -> (79.15, 33.1454)
  line L54 (84.85, 33.1454) -> (82, 34.7909)
  line L55 (96.75, 34.7909) -> (96.75, 28.2091)
  line L56 (82, 28.2091) -> (96.75, 28.2091)
  line L57 (79.15, 33.1454) -> (79.15, 29.8546)
  line L58 (79.15, 29.8546) -> (82, 28.2091)
  line L59 (82, 28.2091) -> (84.85, 29.8546)
  line L60 (70, -62) -> (70, 91.5) construction
  line L61 (82, 91.5) -> (82, -91.5) construction
  line L62 (94, -91.5) -> (94, 91.5) construction
  line L63 (70, -91.5) -> (94, -91.5) construction
  line L64 (84.85, 29.8546) -> (84.85, 33.1454)
  line L65 (82, -8.2091) -> (79.15, -9.8546)
  line L66 (84.85, -9.8546) -> (82, -8.2091)
  line L67 (79.15, -9.8546) -> (79.15, -13.1454)
  line L68 (84.85, -13.1454) -> (84.85, -9.8546)
  line L69 (82, -14.7909) -> (84.85, -13.1454)
  line L70 (79.15, -13.1454) -> (82, -14.7909)
  line L71 (82, -48.2091) -> (79.15, -49.8546)
  line L72 (79.15, -49.8546) -> (79.15, -53.1454)
  line L73 (79.15, -53.1454) -> (82, -54.7909)
  line L74 (82, -8.2091) -> (96.75, -8.2091)
  line L75 (82, -54.7909) -> (84.85, -53.1454)
  line L76 (84.85, -49.8546) -> (82, -48.2091)
  line L77 (84.85, -53.1454) -> (84.85, -49.8546)
  line L78 (96.75, -8.2091) -> (96.75, -14.7909)
  line L79 (82, -14.7909) -> (96.75, -14.7909)
  line L80 (82, -48.2091) -> (96.75, -48.2091)
  line L81 (96.75, -48.2091) -> (96.75, -54.7909)
  line L82 (82, -54.7909) -> (96.75, -54.7909)
  circle A0 centre (82, 71.5) radius 1.7
  circle A1 centre (82, 31.5) radius 1.7
  circle A2 centre (82, -11.5) radius 1.7
  circle A3 centre (82, -51.5) radius 1.7
  circle A4 centre (-82, -51.5) radius 1.7
  circle A5 centre (-82, -11.5) radius 1.7
  circle A6 centre (-82, 31.5) radius 1.7
  circle A7 centre (-82, 71.5) radius 1.7
  point P0 (0, 0)
  point P1 (0, 0)
  point P2 (-82, 71.5)
  point P3 (-82, 71.5)
  point P4 (-82, -51.5)
  point P5 (-82, 31.5)
  point P6 (-82, -11.5)
  point P7 (-82, 31.5)
  point P8 (-82, -11.5)
  point P9 (-82, -11.5)
  point P10 (-82, -11.5)
  point P11 (-82, -51.5)
  point P12 (82, 71.5)
  point P13 (82, 31.5)
  point P14 (82, -11.5)
  point P15 (82, -51.5)
  point P16 (82, -51.5)
  point P17 (82, -51.5)
  point P18 (82, -11.5)
  point P19 (82, -11.5)
  point P20 (82, -11.5)
  point P21 (82, -51.5)
  point P22 (82, 31.5)
  point P23 (82, -11.5)
  point P24 (82, -51.5)
  point P25 (-82, -51.5)
  point P26 (-82, -11.5)
  point P27 (-82, 31.5)
  point P28 (-82, 71.5)
  point P29 (-82, 71.5)
  dimension "d233" = 5.7
  dimension "d234" = 12
  dimension "d235" = 12
  dimension "d236" = 20
  dimension "d237" = 40
  dimension "d238" = 40
  dimension "d239" = 40
  dimension "d240" = 5.7
  dimension "d241" = 5.7
  dimension "d242" = 5.7
  dimension "d243" = 3.4
  dimension "d244" = 3.4
  dimension "d245" = 3.4
  dimension "d246" = 3.4
  dimension "d247" = 3.4
  dimension "d248" = 3.4
  dimension "d249" = 3.4
  dimension "d250" = 3.4
  dimension "d255" = 0
  dimension "d256" = 0
  constraints: 166 end point, 8 centre point, 8 point on line, 3 midpoint, 1 coincident, 1 parallel, 1 vertical, 52 other
  measures "d233" distance between parallel lines of L0 L4
  measures "d234" distance between parallel lines of L12 L10
  measures "d235" distance between parallel lines of L10 L13
  measures "d236" distance from line of L9 point (-82, 71.5)
  measures "d237" distance of L10.end point (-82, -51.5)
  measures "d238" distance of point (-82, 31.5) point (-82, 71.5)
  measures "d239" distance of point (-82, -51.5) point (-82, -11.5)
  measures "d240" distance between parallel lines of L15 L19
  measures "d241" distance between parallel lines of L30 L29
  measures "d242" distance between parallel lines of L39 L38
  measures "d243" diameter of A0
  measures "d244" diameter of A1
  measures "d245" diameter of A2
  measures "d246" diameter of A3
  measures "d247" diameter of A4
  measures "d248" diameter of A5
  measures "d249" diameter of A6
  measures "d250" diameter of A7
  measures "d255" distance of point (-82, 71.5) A7.centre
  measures "d256" distance of point (82, 71.5) point (82, 71.5)
extrude "Extrusion31" cut sketch "Skizze46" against normal blind 40 contours A0 | A1 | A2 | A3 | A4 | A5 | A6 | A7
sketch "Skizze47" plane through (89, -91.5, 180.5) normal (0, 0, 1) x (1, 0, 0)
  line L0 (-56.157, 211.6811) -> (19.7468, 211.6811)
  line L1 (19.7468, 211.6811) -> (19.7468, -13.3543)
  line L2 (19.7468, -13.3543) -> (-56.157, -13.3543)
  line L3 (-56.157, -13.3543) -> (-56.157, 211.6811)
  point P0 (-89, 91.5)
  constraints: 8 end point, 2 parallel, 1 horizontal, 1 perpendicular
extrude "Extrusion32" cut sketch "Skizze47" against normal through all
sketch "Skizze48" plane through (-89, -91.5, 24) normal (-1, 0, 0) x (0, 0, 1)
  circle A0 centre (64.5, 95) radius 35.025
  line L0 (64.5, 86.2555) -> (52.4124, 51.1364) construction
  line L1 (89, 95) -> (64.5, 95) construction
  circle A1 centre (64.5, 95) radius 14.195
  line L2 (54.5, 35.25) -> (130, 35.25) projected
  line L3 (54.5, 35.25) -> (64.5, 35.25)
  line L4 (64.5, 35.25) -> (64.5, 95)
  line L5 (64.5, 89.25) -> (54.5, 89.25)
  line L6 (54.5, 95) -> (54.5, 35.25)
  line L7 (156.5, 29.5) -> (0, 29.5) projected
  point P0 (-24, 91.5)
  point P1 (59.5, 35.25)
  dimension "d259" = 70.05
  dimension "d260" = 28.39
  dimension "d261" = 10
  dimension "d262" = 54
  dimension "d292" = 5.75
  constraints: 12 end point, 3 coincident, 2 centre point, 2 horizontal, 2 parallel, 1 midpoint, 1 perpendicular
  measures "d259" diameter of A0
  measures "d260" diameter of A1
  measures "d261" distance between parallel lines of L4 L6
  measures "d262" distance from line of point (59.5, 35.25) L5
  measures "d292" distance between parallel lines of L7 L2
extrude "Extrusion33" cut sketch "Skizze48" against normal up to surface (24 mm away) contours L6 L5 L4 A1 | A1 L4 L5 L6
sketch "Skizze49" plane through (-89, -91.5, 24) normal (-1, 0, 0) x (0, 0, 1)
  circle A0 centre (64.5, 95) radius 35.025
  circle A1 centre (64.5, 100.75) radius 11.25
  arc A2 (50.305, 95) -> (50.305, 95) centre (64.5, 95) ccw projected
  point P0 (-24, 91.5)
  dimension "d265" = 70.05
  dimension "d266" = 22.5
  constraints: 2 centre point, 1 coincident
  measures "d265" diameter of A0
  measures "d266" diameter of A1
extrude "Extrusion34" cut sketch "Skizze49" against normal blind 22 contours A0 | A1 A2 | A1 A2 | A2 A1
sketch "Skizze53" plane through (-65, -32.25, 154) normal (1, 0, 0) x (0, 0, -1)
  circle A0 centre (65.5, 35.75) radius 14.195 projected
  circle A1 centre (65.5, 35.75) radius 11.25
  point P0 (154, 32.25)
  constraints: 1 centre point, 1 coincident
sketch "Skizze54" plane through (-89, -91.5, 24) normal (-1, 0, 0) x (0, 0, 1)
  circle A0 centre (86.9506, 117.4506) radius 3
  circle A1 centre (86.9506, 117.4506) radius 5
  circle A2 centre (64.5, 95) radius 11.25
  circle A3 centre (64.5, 95) radius 11.25
  circle A4 centre (42.0494, 117.4506) radius 5
  circle A5 centre (42.0494, 72.5494) radius 5
  circle A6 centre (86.9506, 72.5494) radius 5
  circle A7 centre (64.5, 95) radius 11.25
  circle A8 centre (64.5, 95) radius 14.195 projected
  point P0 (-24, 91.5)
  dimension "d295" = 10
  dimension "d296" = 360
  constraints: 8 centre point, 4 coincident, 9 other
  measures "d295" diameter of A1
extrude "Extrusion38" cut sketch "Skizze54" against normal through all contours A0 | A1 | A4 | A5 | A6
chamfer "Fasen2" distance 1.5 angle 45 4 edges at (-65, 25.9506, 61.0494) (-65, 25.9506, 105.9506) (-65, -18.9506, 105.9506) (-65, -18.9506, 61.0494)
sketch "Skizze55" plane through (-89, -91.5, 24) normal (-1, 0, 0) x (0, 0, 1)
  circle A0 centre (64.5, 95) radius 11.25
  line L0 (37.2764, 120.1023) -> (39.3977, 122.2236)
  line L1 (91.7236, 69.8977) -> (89.6023, 67.7764)
  line L2 (89.6023, 67.7764) -> (37.2764, 120.1023)
  line L3 (39.3977, 122.2236) -> (91.7236, 69.8977)
  line L4 (100.6275, 86.8726) -> (99.851, 83.9748)
  line L5 (28.3725, 103.1274) -> (29.149, 106.0252)
  line L6 (29.149, 106.0252) -> (100.6275, 86.8726)
  line L7 (99.851, 83.9748) -> (28.3725, 103.1274)
  line L8 (99.851, 106.0252) -> (100.6275, 103.1274)
  line L9 (29.149, 83.9748) -> (28.3725, 86.8726)
  line L10 (28.3725, 86.8726) -> (99.851, 106.0252)
  line L11 (100.6275, 103.1274) -> (29.149, 83.9748)
  line L12 (89.6023, 122.2236) -> (91.7236, 120.1023)
  line L13 (39.3977, 67.7764) -> (37.2764, 69.8977)
  line L14 (37.2764, 69.8977) -> (89.6023, 122.2236)
  line L15 (91.7236, 120.1023) -> (39.3977, 67.7764)
  line L16 (72.6274, 131.1275) -> (75.5252, 130.351)
  line L17 (56.3726, 58.8725) -> (53.4748, 59.649)
  line L18 (53.4748, 59.649) -> (72.6274, 131.1275)
  line L19 (75.5252, 130.351) -> (56.3726, 58.8725)
  line L20 (53.4748, 130.351) -> (56.3726, 131.1275)
  line L21 (75.5252, 59.649) -> (72.6274, 58.8725)
  line L22 (72.6274, 58.8725) -> (53.4748, 130.351)
  line L23 (56.3726, 131.1275) -> (75.5252, 59.649)
  line L24 (37.2764, 120.1023) -> (39.3977, 122.2236)
  line L25 (91.7236, 69.8977) -> (89.6023, 67.7764)
  line L26 (89.6023, 67.7764) -> (37.2764, 120.1023)
  line L27 (39.3977, 122.2236) -> (91.7236, 69.8977)
  line L28 (28.3725, 103.1274) -> (29.149, 106.0252)
  line L29 (100.6275, 86.8726) -> (99.851, 83.9748)
  line L30 (99.851, 83.9748) -> (28.3725, 103.1274)
  line L31 (29.149, 106.0252) -> (100.6275, 86.8726)
  line L32 (29.149, 83.9748) -> (28.3725, 86.8726)
  line L33 (99.851, 106.0252) -> (100.6275, 103.1274)
  line L34 (100.6275, 103.1274) -> (29.149, 83.9748)
  line L35 (28.3725, 86.8726) -> (99.851, 106.0252)
  line L36 (39.3977, 67.7764) -> (37.2764, 69.8977)
  line L37 (89.6023, 122.2236) -> (91.7236, 120.1023)
  line L38 (91.7236, 120.1023) -> (39.3977, 67.7764)
  line L39 (37.2764, 69.8977) -> (89.6023, 122.2236)
  line L40 (56.3726, 58.8725) -> (53.4748, 59.649)
  line L41 (72.6274, 131.1275) -> (75.5252, 130.351)
  line L42 (75.5252, 130.351) -> (56.3726, 58.8725)
  line L43 (53.4748, 59.649) -> (72.6274, 131.1275)
  line L44 (75.5252, 59.649) -> (72.6274, 58.8725)
  line L45 (53.4748, 130.351) -> (56.3726, 131.1275)
  line L46 (56.3726, 131.1275) -> (75.5252, 59.649)
  line L47 (72.6274, 58.8725) -> (53.4748, 130.351)
  circle A1 centre (64.5, 95) radius 14.195 projected
  point P0 (-24, 91.5)
  point P1 (63.4393, 93.9393)
  point P2 (64.5, 95)
  point P3 (65.5607, 96.0607)
  point P4 (64.8882, 96.4489)
  point P5 (64.5, 95)
  point P6 (64.1118, 93.5511)
  point P7 (64.1118, 96.4489)
  point P8 (64.5, 95)
  point P9 (64.8882, 93.5511)
  point P10 (63.4393, 96.0607)
  point P11 (64.5, 95)
  point P12 (65.5607, 93.9393)
  point P13 (63.0511, 95.3882)
  point P14 (64.5, 95)
  point P15 (65.9489, 94.6118)
  point P16 (63.0511, 94.6118)
  point P17 (64.5, 95)
  point P18 (65.9489, 95.3882)
  point P19 (63.4393, 93.9393)
  point P20 (64.5, 95)
  point P21 (65.5607, 96.0607)
  point P22 (64.1118, 93.5511)
  point P23 (64.5, 95)
  point P24 (64.8882, 96.4489)
  point P25 (64.8882, 93.5511)
  point P26 (64.5, 95)
  point P27 (64.1118, 96.4489)
  point P28 (65.5607, 93.9393)
  point P29 (64.5, 95)
  point P30 (63.4393, 96.0607)
  point P31 (65.9489, 94.6118)
  point P32 (64.5, 95)
  point P33 (63.0511, 95.3882)
  point P34 (65.9489, 95.3882)
  point P35 (64.5, 95)
  point P36 (63.0511, 94.6118)
  point P37 (64.5, 89.2044)
  point P38 (66.6213, 92.8787)
  point P39 (70.2956, 95)
  point P40 (66.6213, 97.1213)
  point P41 (64.5, 100.7956)
  point P42 (56.3726, 131.1275)
  point P43 (62.3787, 97.1213)
  point P44 (58.7044, 95)
  point P45 (62.3787, 92.8787)
  dimension "d304" = 360
  constraints: 96 end point, 15 coincident, 2 midpoint, 2 parallel, 1 centre point, 1 perpendicular, 155 other
extrude "Extrusion39" cut sketch "Skizze55" against normal up to surface (22 mm away) contours L11 L6 L15 L10 A0 | A0 L10 A1 L11 | L6 A1 L7 A0 | A0 L7 L3 L11 L6 | A1 L10 L8 L11 | L11 L3 L15 L6 | L6 L4 L7 A1 | L15 L6 L19 L10 | L15 L3 L19 L6 | L11 L23 L15 L3 | L3 L7 L23 L11 | L19 L6 L23 L10 | L10 L23 L14 L19 | L19 L3 L23 L6 | L15 L23 L19 L3 | L23 L7 L19 L11 | L11 L19 L15 L23 | L23 L2 L19 L7 | L19 L14 L23 L18 A0 | A0 L18 A1 L19 | L23 L6 L3 L10 | L10 L3 L14 L23 | L23 L3 L6 | L19 L23 L3 | L15 L19 L23 | L19 L7 L15 L11 | L11 L15 L19 | L23 A1 L22 A0 | A0 L22 L19 L2 L23 | L19 L2 L15 L7 | A1 L18 L16 L19 | L14 L3 L18 L23 | L10 L6 L14 L3 | L3 L6 L10 | L3 L23 L19 L15 L11 L7 L2 L22 L18 L14 L10 L6 | L15 L7 L11 | L23 L21 L22 A1 | L19 L22 L15 L2 | L15 L2 L11 L7 | L23 L18 L3 L22 A0 | A0 L22 A1 L23 | L14 L6 L18 L3 | L10 L14 L6 | L11 L2 L7 | L19 A1 L18 A0 | A0 L18 L15 L22 L19 | L15 L22 L11 L2 | A1 L22 L20 L23 | L18 L6 L22 L3 | L14 L10 L18 L6 | L14 L18 L10 | L7 L22 L2 | L2 L11 L22 L7 | L19 L17 L18 A1 | L15 L18 L11 L22 | L18 L10 L22 L6 | L18 L14 L22 L10 | L18 L22 L14 | L22 L7 L18 L2 | L2 L18 L22 | L22 L11 L18 L7 | L22 L10 L2 L6 | L22 L14 L2 L10 | L22 L18 L2 L14 | L18 L7 L14 L2 | L18 L11 L14 L7 | L6 L2 L10 L7 A0 | A0 L7 A1 L6 | L2 L14 L7 L10 | L14 L11 A0 L10 L7 | L11 A1 L10 A0 | A1 L7 L5 L6 | L11 L9 L10 A1
sketch "Skizze56" plane through (-89, -91.5, 24) normal (-1, 0, 0) x (0, 0, 1)
  circle A0 centre (64.5, 95) radius 11.25
  circle A1 centre (64.5, 125) radius 6
  circle A2 centre (64.5, 65) radius 6
  arc A3 (53.9943, 128.4123) -> (42.694, 122.4089) centre (64.5, 95) ccw projected
  point P0 (-24, 91.5)
  dimension "d307" = 12
  dimension "d308" = 12
  dimension "d309" = 30
  dimension "d310" = 30
  constraints: 3 centre point, 2 coincident
  measures "d307" diameter of A1
  measures "d308" diameter of A2
  measures "d309" distance of point (64.5, 95) A1.centre
  measures "d310" distance of point (64.5, 95) A2.centre
extrude "Extrusion40" cut sketch "Skizze56" against normal through all contours A1 | A2
sketch "Skizze60" plane through (-68, 91.5, 178.5) normal (0, 1, 0) x (1, 0, 0)
  line L0 (0, 24.5) -> (3, 24.5)
  line L1 (3, 24.5) -> (3, 47.5)
  line L2 (3, 47.5) -> (0, 47.5)
  line L3 (0, 47.5) -> (0, 24.5)
  point P0 (68, 178.5)
  dimension "d347" = 3
  dimension "d348" = 23
  constraints: 8 end point, 2 parallel, 1 horizontal, 1 perpendicular
  measures "d347" distance of L2.end L1.end
  measures "d348" distance of L1.end L0.end
extrude "Extrusion42" cut sketch "Skizze60" against normal blind 50
sketch "Skizze61" plane through (-77, 91.5, 89.5) normal (0, 1, 0) x (1, 0, 0)
  line L0 (12, -41.5) -> (9, -41.5) projected
  line L1 (12, -64.5) -> (12, 11) projected
  line L2 (9, -41.5) -> (12, -41.5)
  line L3 (12, -41.5) -> (12, -64.5)
  line L4 (12, -64.5) -> (9, -64.5)
  line L5 (9, -64.5) -> (9, -41.5)
  point P0 (77, 89.5)
  constraints: 8 end point, 2 parallel, 1 horizontal, 1 perpendicular
extrude "Extrusion43" add sketch "Skizze61" against normal blind 3
mirror "Spiegeln2" about plane through (0, 0, 0) normal (1, 0, 0)
